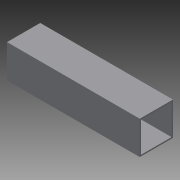
# Autodesk Inventor part: Tube support base 2
Saved by Autodesk Inventor 2015 (Build 190159000, 159)
## iProperties
Created: 2016-03-22
Part Number: Tube support base 2
Material: Generic
Document SubType Name: Modeling
Designer: Mac
Density: 1 g/cm^3
Appearance: Default
Author: Mac
Autodesk Inventor part; units mm, degrees
ref_plane "YZ Plane" through (0, 0, 0) normal (1, 0, 0) x (0, 1, 0)
ref_plane "XZ Plane" through (0, 0, 0) normal (0, 1, 0) x (-1, 0, 0)
ref_plane "XY Plane" through (0, 0, 0) normal (0, 0, 1) x (1, 0, 0)
sketch "Sketch1" plane through (0, 0, 0) normal (1, 0, 0) x (0, 1, 0)
  line L0 (25.4, 25.4) -> (-25.4, 25.4)
  line L1 (-25.4, 25.4) -> (-25.4, -25.4)
  line L2 (-25.4, -25.4) -> (25.4, -25.4)
  line L3 (25.4, -25.4) -> (25.4, 25.4)
  line L4 (-23.2918, 23.2918) -> (23.2918, 23.2918)
  line L5 (23.2918, 23.2918) -> (23.2918, -23.2918)
  line L6 (23.2918, -23.2918) -> (-23.2918, -23.2918)
  line L7 (-23.2918, -23.2918) -> (-23.2918, 23.2918)
  point P0 (0, 0)
  point P1 (23.2918, 0)
  point P2 (0, -23.2918)
  dimension "d0" = 50.8
  dimension "d1" = 50.8
  dimension "d2" = 2.1082
  constraints: 16 end point, 4 parallel, 2 midpoint, 2 perpendicular, 1 horizontal, 1 horizontal alignment, 1 vertical alignment, 3 other
  measures "d0" distance of L2.end L0.start
  measures "d1" distance of L1.end L2.end
  measures "d2" distance between parallel lines of L5 L3
extrude "Extrusion1" add sketch "Sketch1" along normal mid plane 203.2
body "Solid1"
